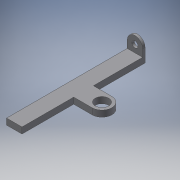
# Autodesk Inventor part: frame
Saved by Autodesk Inventor 2017 (Build 210142000, 142)
## iProperties
Created: 2018-01-02
Part Number: frame
Material: Generic
Document SubType Name: Modeling
Designer: RLanting
Density: 1 g/cm^3
Appearance: Default
Author: RLanting
Autodesk Inventor part; units mm, degrees
ref_plane "YZ Plane" through (0, 0, 0) normal (1, 0, 0) x (0, 1, 0)
ref_plane "XZ Plane" through (0, 0, 0) normal (0, 1, 0) x (-1, 0, 0)
ref_plane "XY Plane" through (0, 0, 0) normal (0, 0, 1) x (1, 0, 0)
sketch "Sketch1" plane through (0, 0, 0) normal (0, 0, 1) x (1, 0, 0)
  circle A0 centre (0, 0) radius 11
  line L0 (0, 0) -> (-30, 0) construction
  line L1 (0, 16) -> (-30, 16)
  line L2 (-30, -16) -> (0, -16)
  arc A1 (0, -16) -> (0, 16) centre (0, 0) ccw
  arc A2 (-30, 16) -> (-30, -16) centre (-30, 0) ccw construction
  line L3 (-30, 16) -> (-30, -16)
  line L4 (-30, 130) -> (-55, 130)
  line L5 (-55, 130) -> (-55, -130)
  line L6 (-55, -130) -> (-30, -130)
  line L7 (-30, -130) -> (-30, 130)
  point P0 (-15, 0)
  point P1 (-30, 0)
  dimension "d0" = 22
  dimension "d1" = 5
  dimension "d2" = 30
  dimension "d3" = 260
  dimension "d4" = 25
  constraints: 18 end point, 4 point on circle, 4 tangent, 3 centre point, 3 midpoint, 3 parallel, 2 horizontal, 1 coincident, 1 perpendicular, 1 vertical
  measures "d0" diameter of A0
  measures "d1" radial gap between concentric circles of A0 A1
  measures "d2" distance of L0.start L0.end
  measures "d3" distance of L4.end L5.end
  measures "d4" distance of L4.start L4.end
extrude "Extrusion1" add sketch "Sketch1" along normal blind 10
sketch "Sketch2" plane through (-55, 130, 0) normal (0, 1, 0) x (1, 0, 0)
  line L0 (25, -10) -> (0, -10) construction
  line L1 (12.5, -10) -> (12.5, -22) construction
  circle A0 centre (12.5, -22) radius 5
  line L2 (12.5, -10) -> (12.5, -22) construction
  line L3 (25, -10) -> (25, -22)
  line L4 (0, -22) -> (0, -10)
  arc A1 (25, -10) -> (0, -10) centre (12.5, -10) ccw construction
  arc A2 (0, -22) -> (25, -22) centre (12.5, -22) ccw
  line L5 (0, -10) -> (25, -10)
  point P0 (55, 0)
  point P1 (12.5, -16)
  dimension "d7" = 10
  dimension "d8" = 12
  constraints: 12 end point, 4 point on circle, 4 tangent, 3 centre point, 3 equal length, 2 midpoint, 1 coincident, 1 vertical
  measures "d7" diameter of A0
  measures "d8" distance of L1.start L1.end
extrude "Extrusion2" add sketch "Sketch2" against normal blind 4
sketch "Sketch3" plane through (0, 0, 10) normal (0, 0, 1) x (1, 0, 0)
  line L0 (-55, 130) -> (-55, -130) projected
  line L1 (-55, -130) -> (-30, -130) projected
  line L2 (-55, -130) -> (-30, -130)
  line L3 (-30, -130) -> (-30, -30)
  line L4 (-30, -30) -> (-55, -30)
  line L5 (-55, -30) -> (-55, -130)
  point P0 (0, 0)
  dimension "d11" = 100
  constraints: 8 end point, 3 equal length, 1 perpendicular
  measures "d11" distance between parallel lines of L1 L4
extrude "Extrusion3" cut sketch "Sketch3" against normal through all
sketch "Sketch4" plane through (0, 0, 10) normal (0, 0, 1) x (1, 0, 0)
  line L0 (-55, -30) -> (-49, -30)
  line L1 (-49, -30) -> (-49, 126)
  line L2 (-49, 126) -> (-55, 126)
  line L3 (-55, 126) -> (-55, -30)
  line L4 (-55, 126) -> (-30, 126) projected
  line L5 (-49, 3) -> (-49, -97) construction
  point P0 (0, 0)
  dimension "d18" = 6
  constraints: 10 end point, 2 parallel, 2 point on line, 1 horizontal, 1 perpendicular
  measures "d18" distance of L0.start L0.end
extrude "Extrusion4" add sketch "Sketch4" along normal blind 5.1
sketch "Sketch5" plane through (-55, 126, 0) normal (0, -1, 0) x (1, 0, 0)
  line L0 (5.5, 23.8249) -> (5.5, 20.1751) construction
  line L1 (0, 15.1) -> (6, 15.1) projected
  line L2 (0, 15.1) -> (5.5, 15.1)
  line L3 (5.5, 15.1) -> (5.5, 22)
  line L4 (5.5, 22) -> (0, 22)
  line L5 (0, 22) -> (0, 15.1)
  line L6 (5.5, 22) -> (5.5, 32.3562)
  arc A0 (25, 22) -> (0, 22) centre (12.5, 22) ccw projected
  arc A1 (5.5, 32.3562) -> (0, 22) centre (12.5, 22) ccw
  line L7 (5.5, 22) -> (0, 22)
  point P0 (55, 0)
  constraints: 12 end point, 3 point on circle, 2 coincident, 2 horizontal, 2 parallel, 1 centre point, 1 midpoint, 1 perpendicular, 1 vertical
extrude "Extrusion5" add sketch "Sketch5" along normal blind 10
sketch "Sketch6" plane through (0, 0, 0) normal (0, 0, -1) x (-1, 0, 0)
  line L0 (30, 130) -> (-15.0463, 5.4414)
  arc A0 (0, 16) -> (0, -16) centre (0, 0) ccw projected
  arc A1 (0, 16) -> (-15.0463, 5.4414) centre (0, 0) ccw
  line L1 (0, 16) -> (30, 16) projected
  line L2 (0, 16) -> (30, 16)
  line L3 (30, 16) -> (30, 130) projected
  line L4 (30, 16) -> (30, 130)
  constraints: 6 end point, 3 point on circle, 1 centre point, 1 coincident, 1 collinear, 1 perpendicular, 1 tangent
extrude "Extrusion6" add sketch "Sketch6" against normal up to surface (10 mm away)
sketch "Sketch7" plane through (0, 0, 10) normal (0, 0, 1) x (1, 0, 0)
  line L0 (-20, 50) -> (-20, 70) construction
  circle A0 centre (-20, 50) radius 2.5
  circle A1 centre (-20, 70) radius 2.5
  line L1 (-55, 116) -> (-55, -30) projected
  line L2 (-30, 130) -> (-55, 130) projected
  point P0 (0, 0)
  dimension "d21" = 5
  dimension "d22" = 20
  dimension "d23" = 35
  dimension "d24" = 80
  constraints: 2 centre point, 2 coincident, 2 end point, 1 equal radius, 1 vertical
  measures "d21" diameter of A0
  measures "d22" distance of L0.start L0.end
  measures "d23" distance between parallel lines of L1 L0
  measures "d24" distance from line of L2 L0.start
extrude "Extrusion7" cut sketch "Sketch7" against normal through all
body "Solid1"
